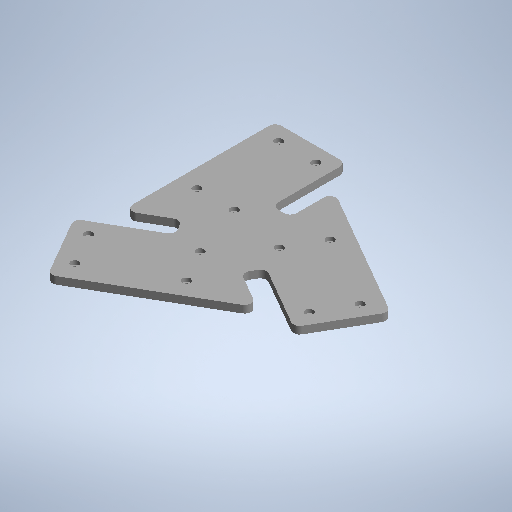
# Autodesk Inventor part: TestBench_Top_Motor_Support
Saved by Autodesk Inventor 2025.4 (Build 294407000, 407)
## iProperties
Created: 2026-05-15
Part Number: TestBench_Top_Motor_Support
Material: Générique
Document SubType Name: Modeling
Designer: louis
Density: 1 g/cm^3
Appearance: Par défaut
Author: louis
Autodesk Inventor part; units mm, degrees
ref_plane "YZ Plane" through (0, 0, 0) normal (1, 0, 0) x (0, 1, 0)
ref_plane "XZ Plane" through (0, 0, 0) normal (0, 1, 0) x (-1, 0, 0)
ref_plane "XY Plane" through (0, 0, 0) normal (0, 0, 1) x (1, 0, 0)
sketch "Sketch2" plane through (0, 0, 0) normal (0, 0, 1) x (1, 0, 0)
  line L0 (-50, 83) -> (-50, 17) construction
  line L1 (-50, 17) -> (-20, 17) construction
  line L2 (-20, 17) -> (-20, 83) construction
  line L3 (-20, 83) -> (-50, 83) construction
  line L4 (-50, 83) -> (-20, 17) construction
  line L5 (-50, 17) -> (-20, 83) construction
  line L6 (-7.5, 95) -> (7.5, 95)
  line L7 (7.5, 95) -> (7.5, 5)
  line L8 (7.5, 5) -> (-7.5, 5)
  line L9 (-7.5, 5) -> (-7.5, 95)
  line L10 (-7.5, 95) -> (7.5, 5) construction
  line L11 (7.5, 95) -> (-7.5, 5) construction
  line L12 (-35, 50) -> (0, 50) construction
  line L13 (0, 50) -> (0, 0) construction
  line L14 (-7.5, 35) -> (7.5, 35)
  line L15 (7.5, 35) -> (60.6218, 35)
  circle A0 centre (0, 0) radius 115 construction
  line L16 (0, 0) -> (0, 35)
  line L17 (0, 0) -> (-99.5929, -57.5)
  line L18 (-7.5, 95) -> (-7.5, 114.7552)
  line L19 (-64.8074, -37.4166) -> (-64.8074, 95)
  line L20 (-64.8074, 95) -> (-7.5, 95)
  line L21 (-26.5609, -23.9952) -> (-34.0609, -11.0048)
  line L22 (-86.0224, -41.0048) -> (-8.0801, 3.9952)
  line L23 (-0.5801, -8.9952) -> (-78.5224, -53.9952)
  line L24 (-78.5224, -53.9952) -> (-86.0224, -41.0048)
  line L25 (-8.0801, 3.9952) -> (-0.5801, -8.9952)
  line L26 (34.0609, -11.0048) -> (26.5609, -23.9952)
  line L27 (78.5224, -53.9952) -> (0.5801, -8.9952)
  line L28 (8.0801, 3.9952) -> (86.0224, -41.0048)
  line L29 (86.0224, -41.0048) -> (78.5224, -53.9952)
  line L30 (0.5801, -8.9952) -> (8.0801, 3.9952)
  point P0 (-30.3109, -17.5)
  point P1 (30.3109, -17.5)
  point P2 (-64.8074, -28.7563)
  point P3 (-30.3109, -17.5)
  dimension "d0" = 30
  dimension "d1" = 66
  dimension "d2" = 15
  dimension "d3" = 90
  dimension "d4" = 12.5
  dimension "d5" = 50
  dimension "d6" = 35
  dimension "d15" = 120
  dimension "d16" = 115
  dimension "d31" = 360
  constraints: 62 end point, 7 point on line, 5 coincident, 5 midpoint, 4 parallel, 4 perpendicular, 4 vertical, 3 horizontal, 3 point on circle, 1 centre point, 37 other
  measures "d0" distance of L2.end L0.start
  measures "d1" distance of L1.end L2.end
  measures "d2" distance of L7.end L8.end
  measures "d3" distance of L6.end L7.end
  measures "d4" distance between parallel lines of L2 L9
  measures "d5" distance from line of L13.end L12
  measures "d6" distance from line of L14 L13.end
  measures "d15" angle of L13 L17
  measures "d16" distance of L16.start L17.end
extrude "Extrusion1" add sketch "Sketch2" against normal blind 6 contours L9 L8 L16 L17 L25 L22 L19 L20 | L14 L16 L8 L9 | L22 L25 L17 L21
hole "Hole1" at (-50, 83, 0) at (-20, 83, 0) at (-20, 17, 0) at (-50, 17, 0) direction (0, 0, -1) diameter 3.6 end through all counterbore diameter 6.5 counterbore depth 3 clearance for "Socket Head Cap Screw" size "M3" standard "Ansi Metric M Profile"
pattern_circular "Circular Pattern1" count 3 over 360 about axis through (0, 0, 0) along (0, 0, -1) of "Extrusion1", "Hole1"
fillet "Fillet1" radius 5 15 edges at (114.6761, 8.6249, -3) (86.0224, -41.0048, -3) (-7.5, 95, -3) (-64.8074, 95, -3) (-7.5, 35, -3) (-78.5224, -53.9952, -3) (-26.5609, -23.9952, -3) (-49.8687, -103.6249, -3) (34.0609, -11.0048, -3) (7.5, 70.503, -3) (7.5, 35, -3) (26.5609, -23.9952, -3) (-34.0609, -11.0048, -3) (57.3074, -41.7467, -3) (-64.8074, -28.7563, -3)
body "Solid1"
